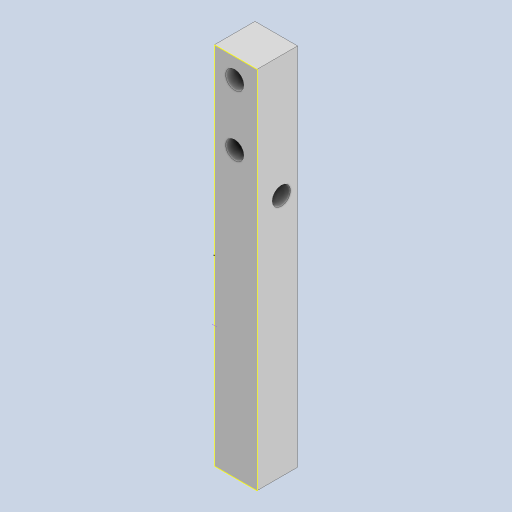
# Autodesk Inventor part: Flange
Saved by Autodesk Inventor 2023.4 (Build 274418000, 418)
## iProperties
Created: 2024-01-12
Part Number: Flange
Material: Generic
Document SubType Name: Modeling
Designer: PalumaCMM
Density: 1 g/cm^3
Appearance: Default
Author: PalumaCMM
Autodesk Inventor part; units mm, degrees
ref_plane "YZ Plane" through (0, 0, 0) normal (1, 0, 0) x (0, 1, 0)
ref_plane "XZ Plane" through (0, 0, 0) normal (0, 1, 0) x (-1, 0, 0)
ref_plane "XY Plane" through (0, 0, 0) normal (0, 0, 1) x (1, 0, 0)
sketch "Sketch1" plane through (0, 0, 0) normal (0, 0, 1) x (1, 0, 0)
  line L0 (0, 0) -> (10.5, 0)
  line L1 (10.5, 0) -> (10.5, 90)
  line L2 (10.5, 90) -> (0, 90)
  line L3 (0, 90) -> (0, 0)
  dimension "d0" = 10.5
  dimension "d1" = 90
  constraints: 8 end point, 2 parallel, 1 horizontal, 1 perpendicular
  measures "d0" distance of L2.end L1.end
  measures "d1" distance of L1.end L0.end
extrude "Extrusion1" add sketch "Sketch1" along normal blind 10
sketch "Sketch4" plane through (0, 0, 10) normal (0, 0, 1) x (1, 0, 0)
  line L0 (0, 90) -> (0, 0) projected
  line L1 (10.5, 0) -> (10.5, 90) projected
  line L2 (10.5, 90) -> (0, 90) projected
  line L3 (0, 0) -> (10.5, 0) projected
  point P0 (0, 30)
  point P1 (0, 45)
  constraints: 1 midpoint, 1 point on line
sketch "Sketch5" plane through (0, 0, 0) normal (-1, 0, 0) x (0, 0, 1)
  circle A0 centre (4, 60) radius 2.5
  line L0 (0, 90) -> (0, 0) projected
  line L1 (0, 90) -> (10, 90) projected
  line L2 (0, 0) -> (10, 0) projected
  point P0 (5, 0)
  point P1 (5, 90)
  dimension "d15" = 5
  dimension "d24" = 4
  dimension "d40" = 30
  constraints: 2 midpoint, 1 centre point, 1 coincident
  measures "d15" diameter of A0
  measures "d24" distance from line of L0 A0.centre
  measures "d40" vertical distance of point (5, 90) point (4, 60)
hole "Hole2" at (0, 60, 4) direction (1, 0, 0) diameter 4.5 end through all clearance for "Countersunk Flat Head Screw ISO 2009/7046" size "M4" standard "ISO"
sketch "Sketch6" plane through (0, 0, 0) normal (0, -1, 0) x (1, 0, 0)
  line L0 (10.5, 6.25) -> (0, 6.25) projected
  line L1 (0, 0) -> (10.5, 0) construction
  line L2 (10.5, 0) -> (10.5, 10) construction
  line L3 (0, 10) -> (10.5, 10) construction
  line L4 (0, 0) -> (0, 10) construction
  point P0 (5.25, 5)
  dimension "d26" = 10
  dimension "d27" = 10.5
  dimension "d29" = 5
  dimension "d30" = 5.25
  measures "d26" distance of L1.start L3.start
  measures "d27" distance of L3.start L2.end
  measures "d29" distance from line of L3 point (5.25, 5)
  measures "d30" distance from line of L4 point (5.25, 5)
hole "Hole3" at (5.25, 0, 5) direction (0, 1, 0) diameter 4.917 depth 17.1 tip angle 118 thread size "M6x1" class "6H" standard "ISO Metric profile"
sketch "Sketch8" plane through (0, 0, 10) normal (0, 0, 1) x (1, 0, 0)
  line L0 (0, 90) -> (0, 0) projected
  line L1 (10.5, 90) -> (0, 90) projected
  point P0 (5, 85)
  point P1 (5, 70)
  dimension "d42" = 5
  dimension "d43" = 5
  dimension "d44" = 5
  dimension "d45" = 15
  measures "d42" distance from line of L0 point (5, 85)
  measures "d43" distance from line of L0 point (5, 70)
  measures "d44" distance from line of L1 point (5, 85)
  measures "d45" distance of point (5, 85) point (5, 70)
hole "Hole4" at (5, 85, 10) at (5, 70, 10) direction (0, 0, -1) diameter 4.5 end through all clearance for "Countersunk Flat Head Screw ISO 2009/7046" size "M4" standard "ISO"
equation "\"d29\" = 0.5 * d26"
equation "\"d30\" = 0.5 * d27"
equation "\"d43\" = d42"
body "Solid1"
